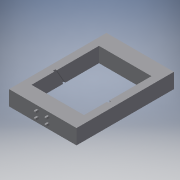
# Autodesk Inventor part: Frame V2
Saved by Autodesk Inventor 2018.3 (Build 223284000, 284)
## iProperties
Created: 2020-11-27
Part Number: Frame V2
Material: Generic
Document SubType Name: Modeling
Designer: daanv
Density: 1 g/cm^3
Appearance: Default
Author: daanv
Autodesk Inventor part; units mm, degrees
ref_plane "YZ Plane" through (0, 0, 0) normal (1, 0, 0) x (0, 1, 0)
ref_plane "XZ Plane" through (0, 0, 0) normal (0, 1, 0) x (-1, 0, 0)
ref_plane "XY Plane" through (0, 0, 0) normal (0, 0, 1) x (1, 0, 0)
sketch "Sketch1" plane through (0, 0, 0) normal (0, 0, 1) x (1, 0, 0)
  line L0 (0, 0) -> (90, 0)
  line L1 (90, 0) -> (90, 130)
  line L2 (90, 130) -> (0, 130)
  line L3 (0, 130) -> (0, 0)
  line L4 (10, 20) -> (80, 20)
  line L5 (80, 20) -> (80, 110)
  line L6 (80, 110) -> (10, 110)
  line L7 (10, 110) -> (10, 20)
  dimension "d0" = 90
  dimension "d1" = 130
  dimension "d2" = 70
  dimension "d3" = 90
  dimension "d16" = 20
  dimension "d17" = 20
  dimension "d18" = 10
  constraints: 16 end point, 4 parallel, 2 horizontal, 2 perpendicular
  measures "d0" distance of L2.end L1.end
  measures "d1" distance of L1.end L0.end
  measures "d2" distance of L6.end L5.end
  measures "d3" distance of L5.end L4.end
  measures "d16" distance between parallel lines of L2 L6
  measures "d17" distance between parallel lines of L0 L4
  measures "d18" distance between parallel lines of L1 L5
extrude "Extrusion1" add sketch "Sketch1" along normal blind 20
sketch "Sketch2" plane through (10, 20, 0) normal (1, 0, 0) x (0, 0, -1)
  line L0 (0, 90) -> (0, 0) projected
  line L1 (0, 42.1132) -> (-20, 30.5662)
  line L2 (-20, 110) -> (-20, -20) projected
  line L3 (0, 42.1132) -> (23.094, 42.1132) construction
  line L4 (-20, 30.5662) -> (-20, 33.5662)
  line L5 (-20, 33.5662) -> (0, 45.1132)
  line L6 (0, 42.1132) -> (0, 45.1132)
  point P0 (-20, 0)
  point P1 (0, -20)
  dimension "d6" = 210
  dimension "d7" = 3
  dimension "d8" = 26.4711
  constraints: 10 end point, 4 point on line, 1 collinear, 1 equal length, 1 horizontal, 1 parallel
  measures "d7" distance of L1.end L4.end
  measures "d8" distance from line of point (-20, 0) L1
extrude "Extrusion2" cut sketch "Sketch2" against normal blind 2
sketch "Sketch3" plane through (80, 20, 0) normal (-1, 0, 0) x (0, 0, 1)
  line L0 (0, 0) -> (0, 90) projected
  line L1 (20, 90) -> (20, 0) projected
  line L2 (0, 42.1132) -> (20, 30.5662)
  line L3 (0, 42.1132) -> (23.094, 42.1132) construction
  line L4 (20, 30.5662) -> (20, 33.5662)
  line L5 (20, 33.5662) -> (0, 45.1132)
  line L6 (0, 42.1132) -> (0, 45.1132)
  point P0 (0, -20)
  dimension "d11" = 30
  dimension "d12" = 3
  dimension "d13" = 26.4711
  constraints: 10 end point, 4 point on line, 1 equal length, 1 horizontal, 1 parallel
  measures "d11" angle of L2 L3
  measures "d12" distance of L2.end L4.end
  measures "d13" distance from line of L1.end L2
extrude "Extrusion3" cut sketch "Sketch3" against normal blind 2
sketch "Sketch4" plane through (0, 0, 0) normal (0, -1, 0) x (1, 0, 0)
  line L0 (0, 0) -> (90, 0) projected
  line L1 (90, 0) -> (90, 20) projected
  line L2 (0, 20) -> (90, 20) projected
  line L3 (0, 0) -> (0, 20) projected
  line L4 (55, 3) -> (35, 3)
  line L5 (35, 3) -> (35, 17)
  line L6 (35, 17) -> (55, 17)
  line L7 (55, 17) -> (55, 3)
  line L8 (53.2053, 7.41) -> (53.87, 5.3643)
  line L9 (53.87, 5.3643) -> (52.1298, 4.1)
  line L10 (52.1298, 4.1) -> (50.3897, 5.3643)
  line L11 (50.3897, 5.3643) -> (51.0543, 7.41)
  line L12 (51.0543, 7.41) -> (53.2053, 7.41)
  line L13 (38.9443, 7.41) -> (39.609, 5.3643)
  line L14 (39.609, 5.3643) -> (37.8689, 4.1)
  line L15 (37.8689, 4.1) -> (36.1287, 5.3643)
  line L16 (36.1287, 5.3643) -> (36.7934, 7.41)
  line L17 (36.7934, 7.41) -> (38.9443, 7.41)
  line L18 (38.9447, 15.55) -> (39.6093, 13.5043)
  line L19 (39.6093, 13.5043) -> (37.8692, 12.24)
  line L20 (37.8692, 12.24) -> (36.129, 13.5043)
  line L21 (36.129, 13.5043) -> (36.7937, 15.55)
  line L22 (36.7937, 15.55) -> (38.9447, 15.55)
  line L23 (53.2053, 15.55) -> (53.87, 13.5043)
  line L24 (53.87, 13.5043) -> (52.1298, 12.24)
  line L25 (52.1298, 12.24) -> (50.3897, 13.5043)
  line L26 (50.3897, 13.5043) -> (51.0543, 15.55)
  line L27 (51.0543, 15.55) -> (53.2053, 15.55)
  point P0 (52.1298, 5.9297)
  point P1 (37.8689, 5.9297)
  point P2 (37.8692, 14.0697)
  point P3 (52.1298, 14.0697)
  dimension "d19" = 20
  dimension "d20" = 14
  dimension "d21" = 3
  dimension "d22" = 3
  dimension "d23" = 35
  dimension "d24" = 35
  dimension "d25" = 1.45
  dimension "d26" = 1.45
  dimension "d27" = 1.1
  dimension "d28" = 1.1
  dimension "d29" = 12.11
  dimension "d30" = 1.13
  dimension "d31" = 1.13
  dimension "d32" = 4.83
  dimension "d33" = 4.83
  dimension "d34" = 1.129
  dimension "d35" = 1.1287
  constraints: 48 end point, 5 horizontal, 3 equal length, 2 parallel, 1 perpendicular, 44 other
  measures "d19" distance of L5.end L6.end
  measures "d20" distance of L4.end L5.end
  measures "d21" distance between parallel lines of L4 L0
  measures "d22" distance between parallel lines of L2 L6
  measures "d23" distance between parallel lines of L1 L7
  measures "d24" distance between parallel lines of L3 L5
  measures "d25" distance between parallel lines of L6 L27
  measures "d26" distance between parallel lines of L22 L6
  measures "d27" distance from line of L4 L9.end
  measures "d28" distance from line of L4 L14.end
  measures "d29" distance of L13.start L11.end
  measures "d30" distance from line of L7 L8.end
  measures "d31" distance from line of L7 L23.end
  measures "d32" distance from line of L12 L24.end
  measures "d33" distance from line of L17 L19.end
  measures "d34" distance from line of L5 L20.end
  measures "d35" distance from line of L5 L15.end
extrude "Extrusion4" add sketch "Sketch4" along normal blind 4 contours L8 L9 L10 L11 L12 | L13 L14 L15 L16 L17 | L18 L19 L20 L21 L22 | L23 L24 L25 L26 L27
chamfer "Chamfer1" distance 0.5 angle 45 20 edges at (52.1298, -4, 15.55) (50.722, -4, 14.5272) (51.2597, -4, 12.8722) (52.9999, -4, 12.8722) (53.5377, -4, 14.5272) (52.1298, -4, 7.41) (53.5377, -4, 6.3872) (52.9999, -4, 4.7322) (51.2597, -4, 4.7322) (50.722, -4, 6.3872) (39.277, -4, 14.5272) (38.7393, -4, 12.8722) (36.9991, -4, 12.8722) (36.4613, -4, 14.5272) (37.8692, -4, 15.55) (37.8689, -4, 7.41) (39.2767, -4, 6.3872) (38.7389, -4, 4.7322) (36.9988, -4, 4.7322) (36.461, -4, 6.3872)
sketch "Sketch5" plane through (0, 130, 0) normal (0, 1, 0) x (1, 0, 0)
  line L0 (90, 0) -> (0, 0) projected
  line L1 (0, 0) -> (0, -20) projected
  line L2 (90, -20) -> (0, -20) projected
  line L3 (90, 0) -> (90, -20) projected
  line L4 (55, -17) -> (35, -17)
  line L5 (35, -17) -> (35, -3)
  line L6 (35, -3) -> (55, -3)
  line L7 (55, -3) -> (55, -17)
  line L8 (52.2861, -15.9) -> (50.4139, -14.8429)
  line L9 (50.4139, -14.8429) -> (50.8408, -12.7357)
  line L10 (50.8408, -12.7357) -> (52.9767, -12.4905)
  line L11 (52.9767, -12.4905) -> (53.87, -14.4461)
  line L12 (53.87, -14.4461) -> (52.2861, -15.9)
  line L13 (37.7119, -15.9) -> (36.128, -14.4461)
  line L14 (36.128, -14.4461) -> (37.0213, -12.4905)
  line L15 (37.0213, -12.4905) -> (39.1572, -12.7357)
  line L16 (39.1572, -12.7357) -> (39.5841, -14.8429)
  line L17 (39.5841, -14.8429) -> (37.7119, -15.9)
  line L18 (37.8674, -7.7585) -> (36.128, -6.4948)
  line L19 (36.128, -6.4948) -> (36.7924, -4.45)
  line L20 (36.7924, -4.45) -> (38.9424, -4.45)
  line L21 (38.9424, -4.45) -> (39.6068, -6.4948)
  line L22 (39.6068, -6.4948) -> (37.8674, -7.7585)
  line L23 (52.1306, -7.7585) -> (50.3912, -6.4948)
  line L24 (50.3912, -6.4948) -> (51.0556, -4.45)
  line L25 (51.0556, -4.45) -> (53.2056, -4.45)
  line L26 (53.2056, -4.45) -> (53.87, -6.4948)
  line L27 (53.87, -6.4948) -> (52.1306, -7.7585)
  circle A0 centre (52.0775, -14.083) radius 1.8289
  circle A1 centre (37.9205, -14.083) radius 1.8289
  circle A2 centre (37.8674, -5.9296) radius 1.8289
  circle A3 centre (52.1306, -5.9296) radius 1.8289
  dimension "d41" = 20
  dimension "d42" = 14
  dimension "d43" = 3
  dimension "d44" = 3
  dimension "d45" = 35
  dimension "d46" = 35
  dimension "d62" = 2.15
  dimension "d63" = 2.15
  dimension "d64" = 2.15
  dimension "d65" = 2.15
  dimension "d66" = 1.13
  dimension "d67" = 1.13
  dimension "d68" = 1.128
  dimension "d69" = 1.1
  dimension "d70" = 1.1
  dimension "d71" = 1.45
  dimension "d72" = 1.45
  dimension "d73" = 1.128
  constraints: 48 end point, 4 coincident, 2 parallel, 2 point on line, 2 vertical alignment, 1 horizontal, 1 perpendicular, 54 other
  measures "d41" distance of L5.end L6.end
  measures "d42" distance of L4.end L5.end
  measures "d43" distance between parallel lines of L2 L4
  measures "d44" distance between parallel lines of L0 L6
  measures "d45" distance between parallel lines of L3 L7
  measures "d46" distance between parallel lines of L1 L5
  measures "d62" distance of L19.end L20.end
  measures "d63" distance of L9.end L10.end
  measures "d64" distance of L14.end L15.end
  measures "d65" distance of L24.end L25.end
  measures "d66" distance from line of L7 L26.end
  measures "d67" distance from line of L7 L11.end
  measures "d68" distance from line of L5 L18.end
  measures "d69" distance from line of L4 L8.start
  measures "d70" distance from line of L4 L13.start
  measures "d71" distance between parallel lines of L6 L25
  measures "d72" distance between parallel lines of L6 L20
  measures "d73" distance from line of L5 L13.end
extrude "Extrusion5" cut sketch "Sketch5" against normal blind 4 contours A0 L8 | L8 L9 L10 L11 L12 | L12 A0 | A0 L9 | L11 A0 | A0 L10 | A1 L13 | L13 L14 L15 L16 L17 | L17 A1 | A1 L14 | L16 A1 | A1 L15 | A2 L18 | L18 L19 L20 L21 L22 | L22 A2 | A2 L19 | L21 A2 | A2 L20 | A3 L23 | L23 L24 L25 L26 L27 | L27 A3 | A3 L24 | L26 A3 | A3 L25
chamfer "Chamfer2" distance 0.5 angle 45 4 edges at (50.2486, 130, 14.083) (36.0916, 130, 14.083) (36.0385, 130, 5.9296) (50.3017, 130, 5.9296)
body "Solid1"
